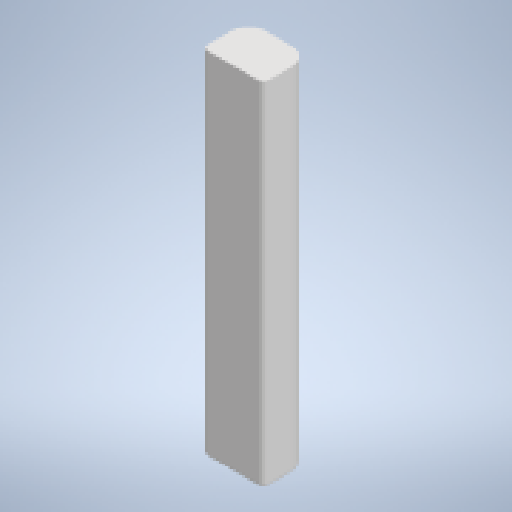
# Autodesk Inventor part: ArmLength
Saved by Autodesk Inventor 2025.2 (Build 292293000, 293)
## iProperties
Created: 2025-02-05
Part Number: ArmLength
Material: Generic
Document SubType Name: Modeling
Designer: andre
Density: 1 g/cm^3
Appearance: Default
Author: andre
Autodesk Inventor part; units mm, degrees
ref_plane "YZ Plane" through (0, 0, 0) normal (1, 0, 0) x (0, 1, 0)
ref_plane "XZ Plane" through (0, 0, 0) normal (0, 1, 0) x (-1, 0, 0)
ref_plane "XY Plane" through (0, 0, 0) normal (0, 0, 1) x (1, 0, 0)
sketch "Sketch1" plane through (0, 0, 0) normal (0, 0, 1) x (1, 0, 0)
  arc A0 (6.6, 0) -> (-2.5948, -6.0685) centre (0, 0) ccw construction
  circle A1 centre (0, 0) radius 6.6
  line L0 (-6.6182, -69.523) -> (6.6182, -69.523)
  line L1 (6.6182, -69.523) -> (6.6182, 69.523)
  line L2 (6.6182, 69.523) -> (-6.6182, 69.523)
  line L3 (-6.6182, 69.523) -> (-6.6182, -69.523)
  line L4 (-6.6182, -69.523) -> (6.6182, 69.523) construction
  line L5 (6.6182, -69.523) -> (-6.6182, 69.523) construction
  line L6 (6.6182, -6.6) -> (-6.6182, -6.6)
  line L7 (-2.8891, -3.8891) -> (2.8891, -3.8891) projected
  arc A2 (2.8891, -3.8891) -> (3.8891, -2.8891) centre (2.8891, -2.8891) ccw projected
  line L8 (3.8891, -2.8891) -> (3.8891, 2.8891) projected
  arc A3 (3.8891, 2.8891) -> (2.8891, 3.8891) centre (2.8891, 2.8891) ccw projected
  line L9 (2.8891, 3.8891) -> (-2.8891, 3.8891) projected
  arc A4 (-2.8891, 3.8891) -> (-3.8891, 2.8891) centre (-2.8891, 2.8891) ccw projected
  line L10 (-3.8891, 2.8891) -> (-3.8891, -2.8891) projected
  arc A5 (-3.8891, -2.8891) -> (-2.8891, -3.8891) centre (-2.8891, -2.8891) ccw projected
  constraints: 14 end point, 2 midpoint, 2 parallel, 2 perpendicular, 2 point on line, 1 centre point, 1 coincident, 1 concentric, 1 horizontal
extrude "Extrusion1" add sketch "Sketch1" along normal blind 10 contours A1 | L6 L3 L2 L1 | A5 L10 A4 L9 A3 L8 A2 L7
fillet "Fillet1" radius 4 2 edges at (6.6182, 31.4615, 0) (-6.6182, 31.4615, 0)
fillet "Fillet2" radius 1 2 edges at (6.6182, 31.4615, 10) (-6.6182, 31.4615, 10)
fillet "Fillet3" radius 1 8 edges at (6.3253, -6.6, 9.7071) (6.6182, -6.6, 6.5) (5.4467, -6.6, 1.1716) (0, -6.6, 0) (-5.4467, -6.6, 1.1716) (-6.6182, -6.6, 6.5) (-6.3253, -6.6, 9.7071) (0, -6.6, 10)
sketch "Sketch2" plane through (0, 0, 0) normal (0, 0, -1) x (-1, 0, 0)
  point P0 (0, 0)
sketch "Sketch3" plane through (0, 0, 0) normal (0, 0, -1) x (-1, 0, 0)
  arc A0 (2.8891, -3.8891) -> (3.8891, -2.8891) centre (2.8891, -2.8891) ccw projected
  line L0 (3.8891, -2.8891) -> (3.8891, 2.8891) projected
  arc A1 (3.8891, 2.8891) -> (2.8891, 3.8891) centre (2.8891, 2.8891) ccw projected
  line L1 (2.8891, 3.8891) -> (-2.8891, 3.8891) projected
  arc A2 (-2.8891, 3.8891) -> (-3.8891, 2.8891) centre (-2.8891, 2.8891) ccw projected
  line L2 (-3.8891, 2.8891) -> (-3.8891, -2.8891) projected
  arc A3 (-3.8891, -2.8891) -> (-2.8891, -3.8891) centre (-2.8891, -2.8891) ccw projected
  line L3 (-2.8891, -3.8891) -> (2.8891, -3.8891) projected
  line L4 (2.5948, -6.0685) -> (-6.6, -10) projected
  line L5 (-6.6, -10) -> (-6.6, 0) projected
  arc A4 (2.5948, -6.0685) -> (-6.6, 0) centre (0, 0) ccw projected
extrude "Extrusion2" cut sketch "Sketch3" against normal blind 5 contours L3 A3 L2 A2 L1 A1 L0 A0
fillet "Fillet4" radius 0.5 20 edges at (-3.5962, -3.5962, 5) (0, -3.8891, 5) (3.5962, -3.5962, 5) (3.8891, 0, 5) (3.5962, 3.5962, 5) (0, 3.8891, 5) (-3.5962, 3.5962, 5) (-3.8891, 0, 5) (2.7537, -3.8891, 0.0023) (3.6288, -3.562, 0.1298) (3.8891, 0, 0.2072) (3.6274, 3.5636, 0.1294) (2.7537, 3.8891, 0.0023) (0, 3.8891, 0) (-2.7537, 3.8891, 0.0023) (-3.6289, 3.5619, 0.1298) (-3.8891, 0, 0.2072) (-3.6286, -3.5622, 0.1297) (-2.7537, -3.8891, 0.0023) (0, -3.8891, 0)
body "Solid1"
